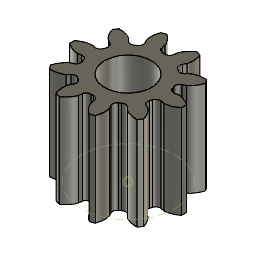
gear_mic (Autodesk Fusion 360 design; units mm, degrees)
part number: 2026-06-01-17-47-26-334
Autodesk Fusion 360 part; units mm, degrees
sketch "Base Circle" plane through (0, 0, 0) normal (0, 0, 1) x (1, 0, 0)
  circle A0 centre (0, 0) radius 3.843
  circle A1 centre (0, 0) radius 2.5
extrude "Extrude3" add sketch "Base Circle" along normal blind 10
sketch "Gear Tooth" plane through (0, 0, 0) normal (0, 0, 1) x (1, 0, 0)
  spline S0 degree 5 poles (4.6331, -0.7809) (4.6369, -0.7816) (4.6445, -0.7827) (4.6559, -0.784) (4.6712, -0.7851) (4.6904, -0.7854) (4.7097, -0.7849) (4.7291, -0.784) (4.7485, -0.7829) (4.7679, -0.7816) (4.7874, -0.7801) (4.8069, -0.7783) (4.8264, -0.7763) (4.8459, -0.7739) (4.8655, -0.7711) (4.8851, -0.768) (4.9048, -0.7646) (4.9244, -0.761) (4.9441, -0.7571) (4.9637, -0.753) (4.9834, -0.7488) (5.0031, -0.7443) (5.0228, -0.7395) (5.0425, -0.7346) (5.0622, -0.7294) (5.0819, -0.7239) (5.1017, -0.7183) (5.1214, -0.7124) (5.1411, -0.7064) (5.1608, -0.7001) (5.1806, -0.6937) (5.2003, -0.6871) (5.22, -0.6802) (5.2397, -0.6732) (5.2594, -0.666) (5.2791, -0.6586) (5.2988, -0.651) (5.3185, -0.6432) (5.3381, -0.6352) (5.3578, -0.6271) (5.3774, -0.6187) (5.3971, -0.6102) (5.4167, -0.6015) (5.4363, -0.5927) (5.4559, -0.5836) (5.4754, -0.5744) (5.495, -0.565) (5.5145, -0.5555) (5.534, -0.5457) (5.5535, -0.5359) (5.573, -0.5258) (5.5924, -0.5156) (5.6119, -0.5052) (5.6313, -0.4946) (5.6506, -0.4839) (5.67, -0.473) (5.6893, -0.4619) (5.7086, -0.4507) (5.7279, -0.4394) (5.7471, -0.4278) (5.7663, -0.4161) (5.7855, -0.4043) (5.8047, -0.3923) (5.8238, -0.3801) (5.8428, -0.3678) (5.8619, -0.3554) (5.8809, -0.3427) (5.8999, -0.33) (5.9188, -0.317) (5.9377, -0.304) (5.9566, -0.2907) (5.9717, -0.28) (5.9829, -0.2719) (5.9904, -0.2665) (5.9942, -0.2638) knots 0 0 0 0 0 0 0.01428571 0.02857143 0.04285714 0.05714286 0.07142857 0.08571429 0.1 0.11428571 0.12857143 0.14285714 0.15714286 0.17142857 0.18571429 0.2 0.21428571 0.22857143 0.24285714 0.25714286 0.27142857 0.28571429 0.3 0.31428571 0.32857143 0.34285714 0.35714286 0.37142857 0.38571429 0.4 0.41428571 0.42857143 0.44285714 0.45714286 0.47142857 0.48571429 0.5 0.51428571 0.52857143 0.54285714 0.55714286 0.57142857 0.58571429 0.6 0.61428571 0.62857143 0.64285714 0.65714286 0.67142857 0.68571429 0.7 0.71428571 0.72857143 0.74285714 0.75714286 0.77142857 0.78571429 0.8 0.81428571 0.82857143 0.84285714 0.85714286 0.87142857 0.88571429 0.9 0.91428571 0.92857143 0.94285714 0.95714286 0.97142857 0.98571429 1 1 1 1 1 1
  spline S1 degree 5 poles (4.6331, 0.7809) (4.6369, 0.7816) (4.6445, 0.7827) (4.6559, 0.784) (4.6712, 0.7851) (4.6904, 0.7854) (4.7097, 0.7849) (4.7291, 0.784) (4.7485, 0.7829) (4.7679, 0.7816) (4.7874, 0.7801) (4.8069, 0.7783) (4.8264, 0.7763) (4.8459, 0.7739) (4.8655, 0.7711) (4.8851, 0.768) (4.9048, 0.7646) (4.9244, 0.761) (4.9441, 0.7571) (4.9637, 0.753) (4.9834, 0.7488) (5.0031, 0.7443) (5.0228, 0.7395) (5.0425, 0.7346) (5.0622, 0.7294) (5.0819, 0.7239) (5.1017, 0.7183) (5.1214, 0.7124) (5.1411, 0.7064) (5.1608, 0.7001) (5.1806, 0.6937) (5.2003, 0.6871) (5.22, 0.6802) (5.2397, 0.6732) (5.2594, 0.666) (5.2791, 0.6586) (5.2988, 0.651) (5.3185, 0.6432) (5.3381, 0.6352) (5.3578, 0.6271) (5.3774, 0.6187) (5.3971, 0.6102) (5.4167, 0.6015) (5.4363, 0.5927) (5.4559, 0.5836) (5.4754, 0.5744) (5.495, 0.565) (5.5145, 0.5555) (5.534, 0.5457) (5.5535, 0.5359) (5.573, 0.5258) (5.5924, 0.5156) (5.6119, 0.5052) (5.6313, 0.4946) (5.6506, 0.4839) (5.67, 0.473) (5.6893, 0.4619) (5.7086, 0.4507) (5.7279, 0.4394) (5.7471, 0.4278) (5.7663, 0.4161) (5.7855, 0.4043) (5.8047, 0.3923) (5.8238, 0.3801) (5.8428, 0.3678) (5.8619, 0.3554) (5.8809, 0.3427) (5.8999, 0.33) (5.9188, 0.317) (5.9377, 0.304) (5.9566, 0.2907) (5.9717, 0.28) (5.9829, 0.2719) (5.9904, 0.2665) (5.9942, 0.2638) knots 0 0 0 0 0 0 0.01428571 0.02857143 0.04285714 0.05714286 0.07142857 0.08571429 0.1 0.11428571 0.12857143 0.14285714 0.15714286 0.17142857 0.18571429 0.2 0.21428571 0.22857143 0.24285714 0.25714286 0.27142857 0.28571429 0.3 0.31428571 0.32857143 0.34285714 0.35714286 0.37142857 0.38571429 0.4 0.41428571 0.42857143 0.44285714 0.45714286 0.47142857 0.48571429 0.5 0.51428571 0.52857143 0.54285714 0.55714286 0.57142857 0.58571429 0.6 0.61428571 0.62857143 0.64285714 0.65714286 0.67142857 0.68571429 0.7 0.71428571 0.72857143 0.74285714 0.75714286 0.77142857 0.78571429 0.8 0.81428571 0.82857143 0.84285714 0.85714286 0.87142857 0.88571429 0.9 0.91428571 0.92857143 0.94285714 0.95714286 0.97142857 0.98571429 1 1 1 1 1 1
  arc A0 (5.9942, -0.2638) -> (5.9942, 0.2638) centre (0, 0) ccw
  line L0 (3.7797, -0.6371) -> (4.6331, -0.7809)
  line L1 (3.7797, 0.6371) -> (4.6331, 0.7809)
  line L2 (3.7797, -0.6371) -> (3.7797, 0.6371)
  point P0 (4.7268, -0.7841)
  point P1 (4.8223, -0.7767)
  point P2 (4.9187, -0.762)
  point P3 (5.0159, -0.7412)
  point P4 (5.1136, -0.7147)
  point P5 (5.2117, -0.6831)
  point P6 (5.31, -0.6465)
  point P7 (5.4084, -0.6052)
  point P8 (5.5068, -0.5592)
  point P9 (5.6051, -0.5088)
  point P10 (5.7031, -0.4539)
  point P11 (5.8006, -0.3948)
  point P12 (5.8977, -0.3314)
  point P13 (4.7268, 0.7841)
  point P14 (4.8223, 0.7767)
  point P15 (4.9187, 0.762)
  point P16 (5.0159, 0.7412)
  point P17 (5.1136, 0.7147)
  point P18 (5.2117, 0.6831)
  point P19 (5.31, 0.6465)
  point P20 (5.4084, 0.6052)
  point P21 (5.5068, 0.5592)
  point P22 (5.6051, 0.5088)
  point P23 (5.7031, 0.4539)
  point P24 (5.8006, 0.3948)
  point P25 (5.8977, 0.3314)
extrude "Extrude4" add sketch "Gear Tooth" along normal blind 10
fillet "Fillet2" radius 0.5 2 edges at (3.7895, -0.6387, 5) (3.7895, 0.6387, 5)
pattern_circular "C-Pattern2" count 10 over 360 about axis through (0, 0, 0) along (0, 0, 1) of "Extrude4", "Fillet2"
sketch "Diametrial Pitch Circle" plane through (0, 0, 0) normal (0, 0, 1) x (1, 0, 0)
  circle A0 centre (0, 0) radius 5 construction
named bodies: "Spur Gear (10 teeth)"
